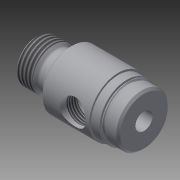
# Autodesk Inventor part: 04R000-0.75_rod_guide
Saved by Autodesk Inventor 2014 SP2 (Build 180246200, 246)
## iProperties
Created: 2019-01-29
Part Number: 04R000-0.75_rod_guide
Material: Generic
Catalog Web Link: www.cadenas.de
Description: Rod Guide-Original Line - Standard Air Cylinders
Vendor: BIMBA
Document SubType Name: Modeling
Designer: psadmin
Manufacturer: BIMBA
Mass: 10.2377 g
Surface Area: 42.5112 cm^2
Volume: 10.2377 cm^3
Density: 1 g/cm^3
Appearance: PSOLRGB-211-211-211
Category: PARTsolutions
Company: BIMBA
Title: 04R000-0.75_rod_guide
Author: Cadenas PARTsolutions
Comments: Original Line - Standard Air Cylinders
PSOL_IDENT_0: {$CADENAS_DATA\23d-libs\bimba\bimba\bimba_imperial\bimba_full_line\original_line_cylinders\standard_
PSOL_IDENT_1: air_cylinders\rod_guide.prj},257 {VTYP=3D},{NB=04R000-0.75_rod_guide},{LINA=04R000-0.75_rod_guide},{
PSOL_IDENT_2: NN=Rod Guide},{DATE=21.03.2018 14:31:21},{GEOMDATE=09.11.2017 12:44:00},{VERSION=},{LINEID=40},{WBVA
PSOL_IDENT_3: R=MNT,ACTING,NR,K,Q,T1,T2,T3,T4,MB,TRIM,CUSH,RODTRANS},{WBNUMERIC=MB,TRIM,CUSH,RODTRANS}  {NB=04R000
PSOL_IDENT_4: -0.75_rod_guide},{LINA=04R000-0.75_rod_guide},{KT=DUMMY},{PN=04R000},{BORE=0.75000000},{BOREPN=04},{
PSOL_IDENT_5: MNT=},{MNTALG='' , 'Front Nose' , 'BF' , 'Front Block' , 'BFT' , 'Front Trunnion' , 'A' , 'Adjustabl
PSOL_IDENT_6: e Stroke'},{ACTING=R},{ACTINGALG= '' , 'Single Acting' , 'R' , 'Reverse/Double Acting' },{NR=},{NRAL
PSOL_IDENT_7: G= '' , 'N/A' },{K=},{Q=},{QALG= '' , 'Without Side Ported Rear Head' , 'Q' , 'With Side Ported Rear
PSOL_IDENT_8: Head' },{T1=},{T2=},{T3=},{T4=},{MB=0},{A1=1.5940},{A1N=0.8750},{A1P=1.5940},{A1B=1.5940},{A2=0.500
PSOL_IDENT_9: 0},{A2N=0.4380},{A2P=0.5000},{A3=0.8440},{A3N=0.1240},{A3P=0.8440},{A4=0.2525},{A4N=0.3130},{A4P=0.2
PSOL_IDENT_10: 525},{A5=0.0300},{A6=0.0000},{A6N=0.1250},{A6P=0.0000},{A7=0.2500},{A7N=0.4390},{A7P=0.2500},{A8=0.0
PSOL_IDENT_11: 100},{A8N=0.0100},{A8NR=0.0300},{D1=0.8625},{D1N=0.8050},{D1P=0.8625},{D1B=0.8325},{D2=0.7615},{D3=0
PSOL_IDENT_12: .0000},{D3N=0.5620},{D3P=0.0000},{D4=0.5310},{D4N=0.2605},{D4P=0.5310},{D4NR=0.3120},{D5=0.2535},{D5
PSOL_IDENT_13: N=0.2535},{D5NR=0.2515},{C1=0.030},{C2=0.0300},{C2N=0.0150},{C2P=0.0300},{C3=0.0000},{C3N=0.0000},{C
PSOL_IDENT_14: 3P=0.0000},{C4=0.0300},{C4N=0.0000},{C4P=0.0300},{NDM=0.6250},{NDMN=0.5000},{NDMP=0.6250},{TAB=UNF},
PSOL_IDENT_15: {D6=0.6225},{D6N=0.6225},{D6P=0.6225},{A9=0.0940},{A9N=0.0940},{A9P=0.0940},{D7=0.5385},{D7N=0.5385}
PSOL_IDENT_16: ,{D7P=0.5385},{A10=0.0855},{A10N=0.0855},{A10P=0.0855},{R1=0.0345},{R1N=0.0345},{R1P=0.0345},{D8=0.5
PSOL_IDENT_17: 310},{D9=0.5000},{D10=0.4405},{A11=0.8030},{A12=0.8970},{A13=1.0220},{A14=0.6250},{A14N=0.6250},{A14
PSOL_IDENT_18: B=0.6250},{D11=0.2500},{D11N=0.2500},{NDM2=0.4050},{NDM2N=0.4050},{NDM2DP=0.2500},{THREAD=0},{HEX=0.
PSOL_IDENT_19: 2535},{HEXN=0.2535},{S1=1.0000},{B1=0.1250},{B2=0.4690},{B22=0.0000},{DB=0.0000},{B3=0.3800},{B4=0.6
PSOL_IDENT_20: 300},{X1=0.0920},{X2=0.6225},{NDM3=0.2500},{NDM4=0.1900},{NDM4DP=0.2500},{DD=1.0000},{CB=0.3280},{CB
PSOL_IDENT_21: DP=0.2190},{PORT=1},{XT=0.4380},{XTX=0.4380},{XT1=0.5000},{XT2=0.3750},{NDMH=0.4375},{OD=0.8075},{ID=
PSOL_IDENT_22: 0.7615},{G=0.0000},{PNUT=0.4060},{TRIM=0},{C11=0.2380},{C22=0.2750},{C33=0.1950},{C44=0.3700},{C55=0
PSOL_IDENT_23: .5350},{CD1=0.1900},{CD2=0.1500},{CD3=0.0725},{CNDM3=0.1380},{CTAB3=UNF},{CUSH=0},{XX=0.63000},{LCD=
PSOL_IDENT_24: 0.0000},{RODTRANS=0.75000}
NN: Rod Guide
NT: Original Line - Standard Air Cylinders
NB: 04R000-0.75_rod_guide
NBSYN: $PN.-$RODTRANS._rod_guide
LINA: 04R000-0.75_rod_guide
BORE: 0
BOREPN: 04
MNT: Front Nose
MNTALG: '' , 'Front Nose' , 'BF' , 'Front Block' , 'BFT' , 'Front Trunnion' , 'A' , 'Adjustable Stroke'
ACTING: Reverse/Double Acting
NR: N/A
K: Standard
Q: Without Side Ported Rear Head
T1: without T1
T2: without T2
T3: without T3
T4: without T4
MB: 0
A1N: 0.875
A1P: 1.594
A1B: 1.594
A2N: 0.438
A2P: 0.5
A3N: 0.124
A3P: 0.844
A4N: 0.313
A4P: 0.2525
A5: 0.03
A6N: 0.125
A6P: 0
A7N: 0.439
A7P: 0.25
A8N: 0.01
A8NR: 0.03
D1N: 0.805
D1P: 0.8625
D1B: 0.8325
D2: 0.7615
D3N: 0.562
D3P: 0
D4N: 0.2605
D4P: 0.531
D4NR: 0.312
D5N: 0.2535
D5NR: 0.2515
C1: 0.03
C2N: 0.015
C2P: 0.03
C3N: 0
C3P: 0
C4N: 0
C4P: 0.03
NDMN: 0.5
NDMP: 0.625
TAB: UNF
D6N: 0.6225
D6P: 0.6225
A9N: 0.094
A9P: 0.094
D7N: 0.5385
D7P: 0.5385
A10N: 0.0855
A10P: 0.0855
R1N: 0.0345
R1P: 0.0345
D8: 0.531
D9: 0.5
D10: 0.4405
A11: 0.803
A12: 0.897
A13: 1.022
A14N: 0.625
A14B: 0.625
D11N: 0.25
NDM2N: 0.405
NDM2DP: 0.25
HEXN: 0.2535
S1: 1
B1: 0.125
B2: 0.469
B22: 0
DB: 0
B3: 0.38
B4: 0.63
X1: 0.092
X2: 0.6225
NDM3: 0.25
NDM4: 0.19
NDM4DP: 0.25
DD: 1
CB: 0.328
CBDP: 0.219
XTX: 0.438
XT1: 0.5
XT2: 0.375
NDMH: 0.4375
TRIM: 0
C11: 0.238
C22: 0.275
C33: 0.195
C44: 0.37
C55: 0.535
CD1: 0.19
CD2: 0.15
CD3: 0.0725
CNDM3: 0.138
CTAB3: UNF
CUSH: 0
LCD: 0
RODTRANS: 0.75
SUPPLIER: BIMBA
ARTICLENO: 04R000-0.75_rod_guide
BOMINFO: 04R000-0.75_rod_guide
CREATOR: CADENAS GmbH
Autodesk Inventor part; units mm, degrees
sketch "Sketch_2" plane through (0, 0, 0) normal (0, 0, 1) x (1, 0, 0)
  line L0 (12.7, 0) -> (0, 0)
  line L1 (0, 0) -> (0, 7.098)
  line L2 (0, 7.098) -> (0.8395, 7.9375)
  line L3 (0.8395, 7.9375) -> (6.6816, 7.9375)
  line L4 (6.6816, 7.9375) -> (7.5202, 7.0965)
  arc A0 (7.5202, 7.0965) -> (8.1407, 6.839) centre (8.1407, 7.7152) ccw
  line L5 (8.1407, 6.839) -> (9.4361, 6.839)
  arc A1 (9.4361, 6.839) -> (10.3124, 7.7153) centre (9.4361, 7.7152) ccw
  line L6 (10.3124, 7.7153) -> (10.3124, 7.9057)
  line L7 (10.3124, 7.9057) -> (12.7, 7.9057)
  line L8 (12.7, 7.9057) -> (12.7, 0)
  line L9 (12.7, 0) -> (0, 0)
  constraints: 20 end point, 4 point on circle, 2 centre point
revolve "Revolution1" add sketch "Sketch_2" angle 360 about axis through (12.7, 0, 0) along (1, 0, 0)
thread "Thread1" size "5/8-18 UNF" class "2A" standard "ANSI Unified Screw Threads" full length
sketch "Sketch_3" plane through (0, 0, 0) normal (0, 0, 1) x (1, 0, 0)
  line L0 (40.4876, 0) -> (12.7, 0)
  line L1 (12.7, 0) -> (12.7, 10.1918)
  line L2 (12.7, 10.1918) -> (13.462, 10.9537)
  line L3 (13.462, 10.9537) -> (34.0741, 10.9537)
  line L4 (34.0741, 10.9537) -> (34.0741, 8.9091)
  line L5 (34.0741, 8.9091) -> (34.8361, 8.9091)
  line L6 (34.8361, 8.9091) -> (35.5981, 9.671)
  line L7 (35.5981, 9.671) -> (39.7256, 9.671)
  line L8 (39.7256, 9.671) -> (40.4876, 8.9091)
  line L9 (40.4876, 8.9091) -> (40.4876, 0)
  line L10 (40.4876, 0) -> (12.7, 0)
  constraints: 22 end point
revolve "Revolution2" add sketch "Sketch_3" angle 360 about axis through (40.4876, 0, 0) along (1, 0, 0)
sketch "Sketch3" plane through (0, 0, 0) normal (-1, 0, 0) x (0, 0, 1)
  point P0 (0, 0)
hole "Hole1" at (0, 0, 0) direction (1, 0, 0) diameter 6.4389 depth 40.4876 countersink diameter 6.9469 countersink angle 90
sketch "Sketch_10" plane through (0, 0, 0) normal (0, 0, 1) x (1, 0, 0)
  line L0 (34.0741, 0) -> (30.8991, 0)
  line L1 (30.8991, 15.3353) -> (30.8991, 10.2553)
  line L2 (30.8991, 10.2553) -> (34.0741, 10.2553)
  line L3 (34.0741, 10.2553) -> (34.0741, 15.3353)
  line L4 (34.0741, 15.3353) -> (30.8991, 15.3353)
  constraints: 10 end point
revolve "Revolution3" cut sketch "Sketch_10" angle 360 about axis through (34.0741, 0, 0) along (1, 0, 0)
sketch "Sketch_40" plane through (0, 0, 0) normal (0, 1, 0) x (-1, 0, 0)
  line L0 (-24.6126, 10.9537) -> (-24.6126, 0)
  line L1 (-24.6126, 0) -> (-27.7876, 0)
  line L2 (-27.7876, 0) -> (-27.7876, 3.1375)
  line L3 (-27.7876, 3.1375) -> (-29.2538, 4.6037)
  line L4 (-29.2538, 4.6037) -> (-29.4521, 10.9537)
  line L5 (-29.4521, 10.9537) -> (-24.6126, 10.9537)
  line L6 (-24.6126, 10.9537) -> (-24.6126, 0)
  constraints: 14 end point
revolve "Revolution4" cut sketch "Sketch_40" angle 360 about axis through (24.6126, 0, 10.9537) along (0, 0, 1)
thread "Thread2" size "1/8" designation "1/8 - 27 NPT" standard "NPT" length 3.8119
sketch "Sketch_47" plane through (0, 0, 0) normal (0, 0, 1) x (1, 0, 0)
  line L0 (34.8361, 0) -> (34.0741, 0)
  line L1 (34.0741, 9.512) -> (34.0741, 8.655)
  line L2 (34.0741, 8.655) -> (34.8361, 8.655)
  line L3 (34.8361, 8.655) -> (34.8361, 8.9091)
  line L4 (34.8361, 8.9091) -> (34.4551, 8.9091)
  line L5 (34.4551, 8.9091) -> (34.1966, 9.1676)
  arc A0 (34.1966, 9.3472) -> (34.1966, 9.1676) centre (34.2864, 9.2574) ccw
  line L6 (34.1966, 9.3472) -> (35.0205, 10.1711)
  line L7 (35.0205, 10.1711) -> (35.0205, 10.2553)
  line L8 (35.0205, 10.2553) -> (34.8173, 10.2553)
  line L9 (34.8173, 10.2553) -> (34.0741, 9.512)
  constraints: 20 end point, 2 point on circle, 1 centre point
revolve "Revolution5" add sketch "Sketch_47" angle 360 about axis through (34.8361, 0, 0) along (1, 0, 0)
ref_plane "dp1_XY" through (12.7, 7.9057, 0) normal (0, 0, 1) x (1, 0, 0)
ref_plane "dp1_YZ" through (12.7, 7.9057, 0) normal (1, 0, 0) x (0, 1, 0)
ref_plane "dp1_ZX" through (12.7, 7.9057, 0) normal (0, 1, 0) x (0, 0, 1)
ref_plane "dp2_XY" through (12.7, -7.9057, 0) normal (0, 0, 1) x (1, 0, 0)
ref_plane "dp2_YZ" through (12.7, -7.9057, 0) normal (1, 0, 0) x (0, 1, 0)
ref_plane "dp2_ZX" through (12.7, -7.9057, 0) normal (0, 1, 0) x (0, 0, 1)
ref_plane "hh_XY" through (0, 7.9375, 0) normal (0, 0, 1) x (1, 0, 0)
ref_plane "hh_YZ" through (0, 7.9375, 0) normal (1, 0, 0) x (0, 1, 0)
ref_plane "hh_ZX" through (0, 7.9375, 0) normal (0, 1, 0) x (0, 0, 1)
ref_plane "port_XY" through (24.6126, 0, 0) normal (0, 0, 1) x (1, 0, 0)
ref_plane "port_YZ" through (24.6126, 0, 0) normal (1, 0, 0) x (0, 1, 0)
ref_plane "port_ZX" through (24.6126, 0, 0) normal (0, 1, 0) x (0, 0, 1)
ref_plane "rod_guide_XY" through (0, 0, 0) normal (1, 0, 0) x (0, 0, -1)
ref_plane "rod_guide_YZ" through (0, 0, 0) normal (0, 0, -1) x (0, 1, 0)
ref_plane "rod_guide_ZX" through (0, 0, 0) normal (0, 1, 0) x (1, 0, 0)
ref_plane "s1_XY" through (10.3124, 0, 0) normal (0, 0, 1) x (1, 0, 0)
ref_plane "s1_YZ" through (10.3124, 0, 0) normal (1, 0, 0) x (0, 1, 0)
ref_plane "s1_ZX" through (10.3124, 0, 0) normal (0, 1, 0) x (0, 0, 1)
ref_plane "s2_XY" through (12.7, 0, 0) normal (0, 0, 1) x (1, 0, 0)
ref_plane "s2_YZ" through (12.7, 0, 0) normal (1, 0, 0) x (0, 1, 0)
ref_plane "s2_ZX" through (12.7, 0, 0) normal (0, 1, 0) x (0, 0, 1)
ref_plane "t1_XY" through (12.7, 0, 0) normal (1, 0, 0) x (0, 0, -1)
ref_plane "t1_YZ" through (12.7, 0, 0) normal (0, 0, -1) x (0, 1, 0)
ref_plane "t1_ZX" through (12.7, 0, 0) normal (0, 1, 0) x (1, 0, 0)
ref_plane "t111_XY" through (12.7, 0, 0) normal (1, 0, 0) x (0, 0, -1)
ref_plane "t111_YZ" through (12.7, 0, 0) normal (0, 0, -1) x (0, 1, 0)
ref_plane "t111_ZX" through (12.7, 0, 0) normal (0, 1, 0) x (1, 0, 0)
ref_plane "to_foot_bracket_XY" through (12.7, 0, 0) normal (1, 0, 0) x (0, 0, -1)
ref_plane "to_foot_bracket_YZ" through (12.7, 0, 0) normal (0, 0, -1) x (0, 1, 0)
ref_plane "to_foot_bracket_ZX" through (12.7, 0, 0) normal (0, 1, 0) x (1, 0, 0)
ref_plane "to_nut_XY" through (10.3124, 0, 0) normal (1, 0, 0) x (0, 0, -1)
ref_plane "to_nut_YZ" through (10.3124, 0, 0) normal (0, 0, -1) x (0, 1, 0)
ref_plane "to_nut_ZX" through (10.3124, 0, 0) normal (0, 1, 0) x (1, 0, 0)
ref_plane "to_rod_XY" through (-19.05, 0, 0) normal (1, 0, 0) x (0, 0, -1)
ref_plane "to_rod_YZ" through (-19.05, 0, 0) normal (0, 0, -1) x (0, 1, 0)
ref_plane "to_rod_ZX" through (-19.05, 0, 0) normal (0, 1, 0) x (1, 0, 0)
ref_plane "to_screw_XY" through (24.6126, 2.032, -6.0452) normal (0, 1, 0) x (1, 0, 0)
ref_plane "to_screw_YZ" through (24.6126, 2.032, -6.0452) normal (1, 0, 0) x (0, 0, -1)
ref_plane "to_screw_ZX" through (24.6126, 2.032, -6.0452) normal (0, 0, -1) x (0, 1, 0)
ref_plane "to_trunnion_brackets_XY" through (11.1252, 0, 0) normal (0, 1, 0) x (1, 0, 0)
ref_plane "to_trunnion_brackets_YZ" through (11.1252, 0, 0) normal (1, 0, 0) x (0, 0, -1)
ref_plane "to_trunnion_brackets_ZX" through (11.1252, 0, 0) normal (0, 0, -1) x (0, 1, 0)
ref_plane "to_trunnion_brackets1_XY" through (11.1252, 12.7, 0) normal (0, 1, 0) x (1, 0, 0)
ref_plane "to_trunnion_brackets1_YZ" through (11.1252, 12.7, 0) normal (1, 0, 0) x (0, 0, -1)
ref_plane "to_trunnion_brackets1_ZX" through (11.1252, 12.7, 0) normal (0, 0, -1) x (0, 1, 0)
ref_plane "to_trunnion_brackets2_XY" through (11.1252, -12.7, 0) normal (0, 1, 0) x (1, 0, 0)
ref_plane "to_trunnion_brackets2_YZ" through (11.1252, -12.7, 0) normal (1, 0, 0) x (0, 0, -1)
ref_plane "to_trunnion_brackets2_ZX" through (11.1252, -12.7, 0) normal (0, 0, -1) x (0, 1, 0)
ref_plane "to_tube_XY" through (34.8361, 0, 0) normal (1, 0, 0) x (0, 0, -1)
ref_plane "to_tube_YZ" through (34.8361, 0, 0) normal (0, 0, -1) x (0, 1, 0)
ref_plane "to_tube_ZX" through (34.8361, 0, 0) normal (0, 1, 0) x (1, 0, 0)
body "Solid1"
